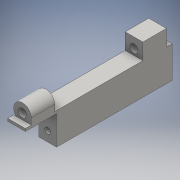
# Autodesk Inventor part: tracks2
Saved by Autodesk Inventor 2016 (Build 200138000, 138)
## iProperties
Created: 2016-04-28
Part Number: tracks2
Material: Generic
Document SubType Name: Modeling
Designer: hesaon
Density: 1 g/cm^3
Appearance: Default
Author: hesaon
Autodesk Inventor part; units mm, degrees
ref_plane "YZ Plane" through (0, 0, 0) normal (1, 0, 0) x (0, 1, 0)
ref_plane "XZ Plane" through (0, 0, 0) normal (0, 1, 0) x (-1, 0, 0)
ref_plane "XY Plane" through (0, 0, 0) normal (0, 0, 1) x (1, 0, 0)
sketch "Sketch8" plane through (0, 0, 0) normal (1, 0, 0) x (0, 1, 0)
  line L0 (0, 0) -> (-50, 0)
  line L1 (-50, 0) -> (-50, -16.325)
  line L2 (-50, -16.325) -> (0, -16.325)
  line L3 (0, -16.325) -> (0, 0)
  dimension "d20" = 50
  dimension "d21" = 16.325
  constraints: 8 end point, 2 parallel, 1 horizontal, 1 perpendicular
  measures "d20" distance of L2.end L1.end
  measures "d21" distance of L1.end L0.end
extrude "Extrusion5" add sketch "Sketch8" along normal blind 6
sketch "Sketch9" plane through (0, -50, -16.325) normal (0, -1, 0) x (1, 0, 0)
  circle A0 centre (3, 12.925) radius 1.4
  circle A1 centre (3, 3.4) radius 1
  line L0 (0, 16.325) -> (6, 16.325) projected
  line L1 (0, 16.325) -> (0, 0) projected
  line L2 (6, 16.325) -> (6, 0) projected
  line L3 (0, 0) -> (6, 0) projected
  line L4 (3, 16.325) -> (3, 0)
  line L5 (0, 8.1625) -> (6, 8.1625)
  dimension "d24" = 2.8
  dimension "d25" = 2
  dimension "d30" = 9.525
  dimension "d31" = 9.525
  dimension "d32" = 0
  dimension "d33" = 0
  constraints: 4 end point, 4 midpoint, 2 centre point
  measures "d24" diameter of A0
  measures "d25" diameter of A1
  measures "d30" diameter of A0.centre L5
  measures "d31" diameter of A1.centre L5
  measures "d32" distance from line of A1.centre L4
  measures "d33" distance from line of A0.centre L4
extrude "Extrusion6" cut sketch "Sketch9" against normal through all contours A0 L4 | L4 A0 | L4 A1 | A1 L4
sketch "Sketch10" plane through (6, 0, 0) normal (1, 0, 0) x (0, 0, -1)
  line L0 (0, 0) -> (0, -50) projected
  line L1 (0, -50) -> (5.5, -50)
  line L2 (5.5, -50) -> (5.5, -48)
  line L3 (5.5, -48) -> (0, -48)
  line L4 (0, -48) -> (0, -50)
  line L5 (16.325, 0) -> (0, 0) projected
  line L6 (0, 0) -> (5.5, 0)
  line L7 (5.5, 0) -> (5.5, -2)
  line L8 (5.5, -2) -> (0, -2)
  line L9 (0, -2) -> (0, 0)
  dimension "d36" = 5.5
  dimension "d37" = 2
  dimension "d38" = 2
  constraints: 16 end point, 4 parallel, 2 horizontal, 2 perpendicular
  measures "d36" distance of L3.end L2.end
  measures "d37" distance of L2.end L1.end
  measures "d38" distance of L6.end L7.end
extrude "Extrusion7" cut sketch "Sketch10" against normal through all
sketch "Sketch11" plane through (6, 0, 0) normal (1, 0, 0) x (0, 0, -1)
  line L0 (0, -2) -> (0, -48) projected
  line L1 (0, -25) -> (16.325, -25)
  line L2 (16.325, -50) -> (16.325, 0) projected
  line L3 (5.5, -40) -> (0, -40)
  line L4 (0, -40) -> (0, -10)
  line L5 (0, -10) -> (5.5, -10)
  line L6 (5.5, -10) -> (5.5, -40)
  line L7 (5.5, -40) -> (0, -10) construction
  line L8 (0, -40) -> (5.5, -10) construction
  point P0 (0, 0)
  point P1 (2.75, -25)
  dimension "d41" = 2.75
  dimension "d42" = 30
  constraints: 14 end point, 4 midpoint, 2 parallel, 2 point on line, 1 horizontal, 1 perpendicular
  measures "d41" distance of L1.start point (2.75, -25)
  measures "d42" distance of L3.end L4.end
extrude "Extrusion8" cut sketch "Sketch11" against normal through all
sketch "Sketch12" plane through (6, -48, -5.5) normal (0, -1, 0) x (1, 0, 0)
  circle A0 centre (-3, 2.1) radius 1.4 projected
  circle A1 centre (-3, 2.1) radius 3
  line L0 (-6, 5.5) -> (-6, 0) projected
  line L1 (0, -10.825) -> (0, 0) projected
  line L2 (-3, -0.9) -> (-6, -0.9)
  line L3 (-6, -10.825) -> (-6, 0) projected
  line L4 (0, 0) -> (0, 5.5) projected
  line L5 (0, 2.1) -> (0, 5.5)
  line L6 (0, 5.5) -> (-6, 5.5)
  line L7 (-6, -0.9) -> (-6, 5.5)
  point P0 (0, -0.9)
  constraints: 8 end point, 2 point on circle, 2 point on line, 2 tangent, 1 centre point, 1 coincident, 1 collinear, 1 horizontal, 1 perpendicular, 1 vertical
extrude "Extrusion9" cut sketch "Sketch12" against normal blind 8 contours L2 L3 L0 A1 | A1 L0 L6 L4
sketch "Sketch13" plane through (0, 0, 0) normal (-1, 0, 0) x (0, 0, 1)
  line L0 (-6.4, -48) -> (-6.4, -40) projected
  line L1 (-16.325, -50) -> (-6.4, -50)
  line L2 (-6.4, -50) -> (-6.4, -39.4)
  line L3 (-6.4, -39.4) -> (-16.325, -39.4)
  line L4 (-16.325, -39.4) -> (-16.325, -50)
  point P0 (0, 0)
  dimension "d47" = 10.6
  constraints: 8 end point, 2 parallel, 1 horizontal, 1 perpendicular
  measures "d47" distance of L2.end L1.end
extrude "Extrusion10" cut sketch "Sketch13" against normal through all
body "Solid2"
